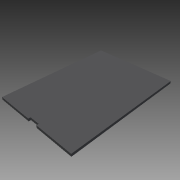
# Autodesk Inventor part: side board
Saved by Autodesk Inventor 2013 (Build 170138000, 138)
## iProperties
Created: 2013-12-08
Part Number: side board
Material: Generic
Document SubType Name: Modeling
Designer: employee
Density: 1 g/cm^3
Author: employee
Autodesk Inventor part; units mm, degrees
ref_plane "YZ Plane" through (0, 0, 0) normal (1, 0, 0) x (0, 1, 0)
ref_plane "XZ Plane" through (0, 0, 0) normal (0, 1, 0) x (-1, 0, 0)
ref_plane "XY Plane" through (0, 0, 0) normal (0, 0, 1) x (1, 0, 0)
sketch "Sketch1" plane through (0, 0, 0) normal (0, 0, 1) x (1, 0, 0)
  line L0 (-197.772, 276.225) -> (197.772, 276.225)
  line L1 (197.772, 276.225) -> (197.772, -276.225)
  line L2 (197.772, -276.225) -> (-197.772, -276.225)
  line L3 (-197.772, -276.225) -> (-197.772, 276.225)
  point P0 (0, 0)
  point P1 (-197.772, 0)
  point P2 (0, 276.225)
  dimension "d0" = 395.544
  dimension "d2" = 552.45
  constraints: 8 end point, 2 midpoint, 2 parallel, 1 horizontal, 1 horizontal alignment, 1 perpendicular, 1 vertical alignment
  measures "d0" distance of L1.end L2.end
  measures "d2" distance of L0.end L1.end
extrude "Extrusion1" add sketch "Sketch1" along normal blind 12.5
sketch "Sketch2" plane through (-197.772, -276.225, 0) normal (0, -1, 0) x (1, 0, 0)
  line L0 (395.544, 0) -> (0, 0) projected
  line L1 (0, 12.5) -> (395.544, 12.5) projected
  circle A0 centre (322.7721, -216.5151) radius 4.1 projected
  circle A1 centre (72.7721, -216.5151) radius 4.1 projected
  circle A2 centre (197.7721, -0.0087) radius 4.1 projected
  arc A3 (204.0221, 10.8166) -> (191.5221, 10.8166) centre (197.7721, -0.0087) ccw projected
  arc A4 (335.2721, -216.5151) -> (204.0221, 10.8166) centre (72.7721, -216.5151) ccw projected
  arc A5 (329.0221, -227.3404) -> (335.2721, -216.5151) centre (322.7721, -216.5151) ccw projected
  arc A6 (66.5221, -227.3404) -> (329.0221, -227.3404) centre (197.7721, -0.0087) ccw projected
  arc A7 (60.2721, -216.5151) -> (66.5221, -227.3404) centre (72.7721, -216.5151) ccw projected
  arc A8 (191.5221, 10.8166) -> (60.2721, -216.5151) centre (322.7721, -216.5151) ccw projected
  line L2 (174.3556, 0) -> (174.3556, 12.5)
  line L3 (221.1887, 0) -> (221.1887, 12.5)
  point P0 (197.772, 0)
  constraints: 4 end point, 4 point on line, 2 point on circle, 1 perpendicular, 1 vertical
extrude "Extrusion2" cut sketch "Sketch2" against normal blind 9.525 contours L0 A2 A8 A3 A4 | A4 A3 A8 L2 L1 L3 | L0 A2 picked at (197.9366, 1.3538)
sketch "Sketch3" plane through (-197.772, -266.7, 0) normal (0, -1, 0) x (1, 0, 0)
  line L0 (221.1887, 0) -> (174.3556, 0) projected
  line L1 (174.3556, 12.5) -> (221.1887, 12.5) projected
  circle A0 centre (197.7721, -0.0087) radius 8 projected
  line L2 (189.7721, 0) -> (189.7721, 12.5)
  line L3 (205.7721, 0) -> (205.7721, 12.5)
  point P0 (197.772, 0)
  point P1 (190.2666, -0.0087)
  point P2 (205.2777, -0.0087)
  constraints: 4 end point, 4 point on line, 2 perpendicular, 2 point on circle, 2 tangent, 2 other
extrude "Extrusion3" cut sketch "Sketch3" against normal blind 7 contours L0 A0 | A0 L2 L1 L3 picked at (198.0933, 3.9197)
body "Solid1"
